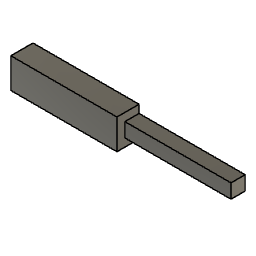
LightSwitcherStraight (Autodesk Fusion 360 design; units mm, degrees)
Autodesk Fusion 360 part; units mm, degrees
sketch "Sketch1" plane through (0, 0, 0) normal (0, 1, 0) x (1, 0, 0)
  line L0 (0, 0) -> (30, 0)
  line L1 (30, 0) -> (30, -8.5)
  line L2 (30, -8.5) -> (0, -8.5)
  line L3 (0, -8.5) -> (0, 0)
  dimension "d1" = 30
  dimension "d2" = 8.5
  constraint horizontal L0
  constraint vertical L1
  constraint horizontal L2
  constraint vertical L3
  constraint coincident L0.start L3.end
  measures "d1" distance of L0.start L0.end
  measures "d2" distance of L0.start L2.end
extrude "Extrude1" add sketch "Sketch1" along normal blind 6.25
sketch "Sketch2" plane through (0, 0, 0) normal (-1, 0, 0) x (0, -1, 0)
  line L0 (0, 0) -> (0, 8.5)
  line L1 (0, 8.5) -> (-6.25, 8.5)
  line L2 (-6.25, 8.5) -> (-6.25, 0)
  line L3 (-6.25, 0) -> (0, 0)
  line L4 (-6.25, 8.5) -> (-4.375, 8.5)
  line L5 (-4.375, 8.5) -> (-4.375, 6.5)
  line L6 (-4.375, 6.5) -> (-1.875, 6.5)
  line L7 (-1.875, 6.5) -> (-1.875, 2)
  line L8 (-1.875, 2) -> (-4.375, 2)
  line L9 (-4.375, 2) -> (-4.375, 6.5)
  dimension "d5" = 1.875
  dimension "d6" = 2
  dimension "d7" = 2.5
  dimension "d8" = 4.5
  constraint coincident L1.end L2.start
  constraint perpendicular L2 L4
  constraint perpendicular L4 L5
  constraint horizontal L6
  constraint vertical L7
  constraint horizontal L8
  constraint vertical L9
  measures "d5" distance of L1.end L4.end
  measures "d6" distance of L4.end L5.end
  measures "d7" distance of L5.end L6.end
  measures "d8" distance of L5.end L8.end
extrude "Extrude2" cut sketch "Sketch2" against normal blind 24 contours L6 L7 L8 L9
sketch "Sketch3" plane through (30, 0, 0) normal (1, 0, 0) x (0, 1, 0)
  line L0 (0, 8.5) -> (0, 0)
  line L1 (0, 0) -> (6.25, 0)
  line L2 (6.25, 0) -> (6.25, 8.5)
  line L3 (6.25, 8.5) -> (0, 8.5)
  line L4 (0, 8.5) -> (2.25, 8.5)
  line L5 (2.25, 8.5) -> (2.25, 6.25)
  line L6 (2.25, 6.25) -> (6.25, 6.25)
  line L7 (6.25, 6.25) -> (6.25, 2.25)
  line L8 (6.25, 2.25) -> (2.25, 2.25)
  line L9 (2.25, 2.25) -> (2.25, 6.25)
  dimension "d11" = 2.25
  dimension "d12" = 2.25
  dimension "d13" = 4
  dimension "d14" = 4
  constraint coincident L0.start L3.end
  constraint horizontal L4
  constraint perpendicular L4 L5
  constraint horizontal L6
  constraint vertical L7
  constraint horizontal L8
  constraint vertical L9
  measures "d11" distance of L0.start L4.end
  measures "d12" distance of L4.end L5.end
  measures "d13" distance of L5.end L6.end
  measures "d14" distance of L5.end L8.end
extrude "Extrude3" add sketch "Sketch3" along normal blind 30 contours L2 L6 L7 L8 L9
